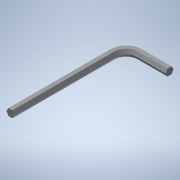
# Autodesk Inventor part: 2mm
Saved by Autodesk Inventor 2022.2 (Build 262287000, 287)
## iProperties
Created: 2012-03-13
Part Number: 2mm
Document SubType Name: Modeling
Designer: jvalasek
Density: 1 g/cm^3
Material: Generic
Appearance: Default
Author: jvalasek
Autodesk Inventor part; units mm, degrees
ref_plane "YZ Plane" through (0, 0, 0) normal (1, 0, 0) x (0, 1, 0)
ref_plane "XZ Plane" through (0, 0, 0) normal (0, 1, 0) x (-1, 0, 0)
ref_plane "XY Plane" through (0, 0, 0) normal (0, 0, 1) x (1, 0, 0)
sketch "Sketch1" plane through (0, 0, 0) normal (0, 1, 0) x (-1, 0, 0)
  line L0 (0.5745, 0.995) -> (1.149, 0)
  line L1 (1.149, 0) -> (0.5745, -0.995)
  line L2 (0.5745, -0.995) -> (-0.5744, -0.995)
  line L3 (-0.5744, -0.995) -> (-1.1489, 0)
  line L4 (-1.1489, 0) -> (-0.5744, 0.995)
  line L5 (-0.5744, 0.995) -> (0.5745, 0.995)
  point P0 (0.0001, 0)
  point P1 (0.5745, 0.995)
  point P2 (1.149, 0)
  point P3 (0.5745, -0.995)
  point P4 (-1.1489, 0)
  point P5 (-0.5744, 0.995)
  point P6 (0.5745, 0.995)
  point P7 (1.149, 0)
  point P8 (0.5745, -0.995)
  point P9 (-1.1489, 0)
  dimension "d1" = 0
  dimension "d0" = 1.99
  constraints: 12 end point, 12 point on line, 5 horizontal, 46 other
  measures "d0" distance between parallel lines of L2 L5
sketch "Sketch2" plane through (0, 0, 0) normal (0, 0, 1) x (1, 0, 0)
  line L0 (-0.0001, 0) -> (-0.0001, 29.6446)
  arc A0 (4.0717, 33.7164) -> (-0.0001, 29.6446) centre (4.0717, 29.6446) ccw
  line L1 (4.0717, 33.7164) -> (12.6439, 33.7164)
  point P0 (-0.5745, 0)
  point P1 (0.5744, 0)
  point P2 (-0.0001, 0)
  dimension "d2" = 1.1489
  dimension "d3" = 33.7164
  dimension "d4" = 12.6439
  dimension "d5" = 4.0718
  constraints: 4 end point, 2 point on circle, 2 tangent, 1 centre point, 1 coincident, 1 perpendicular, 1 vertical
  measures "d2" distance of point (0.574, 0) point (-0.575, 0)
  measures "d3" distance from line of L1 L0.start
  measures "d4" distance from line of L1.end L0
  measures "d5" radius of A0
sweep "Sweep1" add profiles "Sketch1" path "Sketch2"
equation "\"d3\" = 29.346 * d2"
equation "\"d4\" = 11.005 * d2"
equation "\"d5\" = 3.544 * d2"
body "Solid1"
